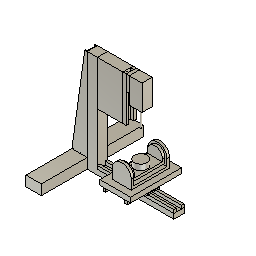
5 Axis CNC Linkage Ideation 3 (Autodesk Fusion 360 design; units mm, degrees)
Autodesk Fusion 360 part; units mm, degrees
sketch "Sketch1" plane through (0, 0, 0) normal (0, 1, 0) x (1, 0, 0)
  line L0 (400, -400) -> (-400, -400)
  line L1 (-400, -400) -> (-400, 400)
  line L2 (-400, 400) -> (400, 400)
  line L3 (400, 400) -> (400, -400)
  line L4 (400, -400) -> (-400, 400) construction
  line L5 (-400, -400) -> (400, 400) construction
  line L6 (-400, -400) -> (-200, -400)
  line L7 (-200, -400) -> (-200, 400)
  line L8 (-200, 400) -> (-400, 400)
  line L9 (-400, 400) -> (-400, -400)
  line L10 (-200, -400) -> (400, -400)
  line L11 (100, -400) -> (100, -50)
  line L12 (100, -50) -> (-200, -50)
  line L13 (200, -400) -> (0, -400)
  line L14 (0, -400) -> (0, -50)
  line L15 (0, -50) -> (200, -50)
  line L16 (200, -50) -> (200, -400)
  line L17 (200, -400) -> (0, -50) construction
  line L18 (0, -400) -> (200, -50) construction
  line L19 (400, 400) -> (-200, 400)
  line L20 (-200, 400) -> (-200, 360)
  line L21 (-200, 360) -> (400, 360)
  line L22 (400, 360) -> (400, 400)
  line L23 (-200, 360) -> (400, 360)
  line L24 (400, 360) -> (400, 335)
  line L25 (400, 335) -> (-200, 335)
  line L26 (-200, 335) -> (-200, 360)
  line L27 (400, 335) -> (-200, 335)
  line L28 (-200, 335) -> (-200, 325)
  line L29 (-200, 325) -> (400, 325)
  line L30 (400, 325) -> (400, 335)
  line L31 (-200, 325) -> (400, 325)
  line L32 (400, 325) -> (400, 300)
  line L33 (400, 300) -> (-200, 300)
  line L34 (-200, 300) -> (-200, 325)
  line L35 (150, -200) -> (50, -200)
  line L36 (50, -200) -> (50, -400)
  line L37 (50, -400) -> (150, -400)
  line L38 (150, -400) -> (150, -200)
  line L39 (150, -200) -> (50, -400) construction
  line L40 (50, -200) -> (150, -400) construction
  line L41 (105, -200) -> (95, -200)
  line L42 (95, -200) -> (95, -50)
  line L43 (95, -50) -> (105, -50)
  line L44 (105, -50) -> (105, -200)
  line L45 (105, -200) -> (95, -50) construction
  line L46 (95, -200) -> (105, -50) construction
  line L47 (175, 260) -> (25, 260)
  line L48 (25, 260) -> (25, 110)
  line L49 (25, 110) -> (175, 110)
  line L50 (175, 110) -> (175, 260)
  line L51 (175, 260) -> (25, 110) construction
  line L52 (25, 260) -> (175, 110) construction
  line L53 (-200, -400) -> (-280, -400)
  line L54 (-280, -400) -> (-280, 400)
  line L55 (-280, 400) -> (-200, 400)
  line L56 (-200, 400) -> (-200, -400)
  line L57 (220, 260) -> (-20, 260)
  line L58 (-20, 260) -> (-20, 300)
  line L59 (-20, 300) -> (220, 300)
  line L60 (220, 300) -> (220, 260)
  line L61 (220, 260) -> (-20, 300) construction
  line L62 (-20, 260) -> (220, 300) construction
  line L63 (25, 300) -> (5, 300)
  line L64 (5, 300) -> (5, 325)
  line L65 (5, 325) -> (25, 325)
  line L66 (25, 325) -> (25, 300)
  line L67 (25, 300) -> (5, 325) construction
  line L68 (5, 300) -> (25, 325) construction
  line L69 (195, 300) -> (175, 300)
  line L70 (175, 300) -> (175, 325)
  line L71 (175, 325) -> (195, 325)
  line L72 (195, 325) -> (195, 300)
  line L73 (195, 300) -> (175, 325) construction
  line L74 (175, 300) -> (195, 325) construction
  line L75 (25, 300) -> (175, 300)
  line L76 (200, 325) -> (0, 325)
  line L77 (0, 325) -> (0, 335)
  line L78 (0, 335) -> (200, 335)
  line L79 (200, 335) -> (200, 325)
  line L80 (200, 325) -> (0, 335) construction
  line L81 (0, 325) -> (200, 335) construction
  line L82 (0, -400) -> (25, -400)
  line L83 (25, -400) -> (25, -50)
  line L84 (25, -50) -> (0, -50)
  line L85 (0, -50) -> (0, -400)
  line L86 (50, -200) -> (25, -200)
  line L87 (25, -200) -> (25, -400)
  line L88 (25, -400) -> (50, -400)
  line L89 (50, -400) -> (50, -200)
  line L90 (25, -400) -> (50, -400)
  line L91 (50, -400) -> (50, -280)
  line L92 (50, -280) -> (25, -280)
  line L93 (25, -280) -> (25, -400)
  line L94 (-280, 400) -> (-400, 400)
  line L95 (-400, 400) -> (-400, 320)
  line L96 (-400, 320) -> (-280, 320)
  line L97 (-280, 320) -> (-280, 400)
  line L98 (25, 260) -> (175, 260)
  line L99 (175, 260) -> (175, 160)
  line L100 (175, 160) -> (25, 160)
  line L101 (25, 160) -> (25, 260)
  point P0 (100, -225)
  point P1 (100, -300)
  point P2 (100, -125)
  point P3 (100, 185)
  point P4 (100, 280)
  point P5 (15, 312.5)
  point P6 (185, 312.5)
  point P7 (100, 330)
  dimension "d1" = 800
  dimension "d2" = 800
  dimension "d3" = 200
  dimension "d4" = 350
  dimension "d5" = 200
  dimension "d6" = 40
  dimension "d7" = 25
  dimension "d8" = 10
  dimension "d9" = 25
  dimension "d10" = 100
  dimension "d11" = 200
  dimension "d12" = 10
  dimension "d13" = 150
  dimension "d14" = 150
  dimension "d15" = 80
  dimension "d21" = 240
  dimension "d22" = 40
  dimension "d27" = 20
  dimension "d28" = 20
  dimension "d29" = 150
  dimension "d30" = 200
  dimension "d41" = 25
  dimension "d46" = 120
  dimension "d55" = 80
  dimension "d73" = 100
  constraint horizontal L0
  constraint perpendicular L0 L1
  constraint parallel L0 L2
  constraint parallel L1 L3
  constraint coincident L4 origin
  constraint coincident L5 origin
  constraint horizontal L6
  constraint vertical L7
  constraint horizontal L8
  constraint vertical L9
  constraint coincident L2 L7.end
  constraint midpoint L10 L11.start
  constraint perpendicular L0 L11
  constraint coincident L7 L12.end
  constraint horizontal L13
  constraint perpendicular L13 L14
  constraint parallel L13 L15
  constraint parallel L14 L16
  constraint coincident L17 P0
  constraint coincident L18 P0
  constraint coincident L10 L13.start
  constraint midpoint L11 P0
  constraint horizontal L19
  constraint vertical L20
  constraint horizontal L21
  constraint vertical L22
  constraint coincident L7 L20.end
  constraint horizontal L23
  constraint vertical L24
  constraint horizontal L25
  constraint vertical L26
  constraint coincident L3 L24.end
  constraint horizontal L27
  constraint vertical L28
  constraint horizontal L29
  constraint vertical L30
  constraint coincident L7 L28.end
  constraint horizontal L31
  constraint vertical L32
  constraint horizontal L33
  constraint vertical L34
  constraint coincident L3 L32.end
  constraint horizontal L35
  constraint perpendicular L35 L36
  constraint parallel L35 L37
  constraint parallel L36 L38
  constraint coincident L39 P1
  constraint coincident L40 P1
  constraint coincident L11 P1
  constraint collinear L0 L37
  constraint horizontal L41
  constraint perpendicular L41 L42
  constraint parallel L41 L43
  constraint parallel L42 L44
  constraint coincident L45 P2
  constraint coincident L46 P2
  constraint coincident L11 P2
  constraint collinear L35 L41
  constraint collinear L15 L43
  constraint horizontal L47
  constraint perpendicular L47 L48
  constraint parallel L47 L49
  constraint parallel L48 L50
  constraint coincident L51 P3
  constraint coincident L52 P3
  constraint horizontal L53
  constraint vertical L54
  constraint horizontal L55
  constraint vertical L56
  constraint collinear L12 L15
  constraint collinear L8 L55
  constraint horizontal L57
  constraint perpendicular L57 L58
  constraint parallel L57 L59
  constraint parallel L58 L60
  constraint coincident L61 P4
  constraint coincident L62 P4
  constraint midpoint L33 L59
  constraint midpoint L47 L57
  constraint horizontal L63
  constraint perpendicular L63 L64
  constraint parallel L63 L65
  constraint parallel L64 L66
  constraint coincident L67 P5
  constraint coincident L68 P5
  constraint collinear L59 L63
  constraint collinear L31 L65
  constraint horizontal L69
  constraint perpendicular L69 L70
  constraint parallel L69 L71
  constraint parallel L70 L72
  constraint coincident L73 P6
  constraint coincident L74 P6
  constraint collinear L29 L71
  constraint collinear L33 L69
  constraint perpendicular L70 L75
  constraint midpoint L33 L75
  constraint horizontal L76
  constraint perpendicular L76 L77
  constraint parallel L76 L78
  constraint parallel L77 L79
  constraint coincident L80 P7
  constraint coincident L81 P7
  constraint midpoint L27 L78
  constraint collinear L31 L76
  constraint horizontal L82
  constraint vertical L83
  constraint horizontal L84
  constraint vertical L85
  constraint coincident L15 L83.end
  constraint horizontal L86
  constraint vertical L87
  constraint horizontal L88
  constraint vertical L89
  constraint horizontal L90
  constraint vertical L91
  constraint horizontal L92
  constraint vertical L93
  constraint coincident L36 L91.end
  constraint horizontal L94
  constraint vertical L95
  constraint horizontal L96
  constraint vertical L97
  constraint coincident L9 L95.end
  constraint horizontal L98
  constraint vertical L99
  constraint horizontal L100
  constraint vertical L101
  constraint coincident L50 L99.end
  measures "d1" distance of L1.end L2.end
  measures "d2" distance of L0.end L1.end
  measures "d3" distance of L0.end L6.end
  measures "d4" distance of L11.start L11.end
  measures "d5" distance of L14.end L15.end
  measures "d6" distance of L2.end L21.end
  measures "d7" distance of L20.end L25.end
  measures "d8" distance of L24.end L29.end
  measures "d9" distance of L28.end L33.end
  measures "d10" distance of L36.end L37.end
  measures "d11" distance of L35.end L36.end
  measures "d12" distance of L42.end L43.end
  measures "d13" distance of L48.end L49.end
  measures "d14" distance of L47.end L48.end
  measures "d15" distance of L6.end L53.end
  measures "d21" distance of L58.end L59.end
  measures "d22" distance of L57.start L59.end
  measures "d27" distance of L64.end L65.end
  measures "d28" distance of L70 L72
  measures "d29" distance of L63.start L69.end
  measures "d30" distance of L77.end L78.end
  measures "d41" distance of L13.end L82.end
  measures "d46" distance of L82.end L92.end
  measures "d55" distance of L54.end L96.end
  measures "d73" distance of L47.end L100.end
extrude "Extrude1" add sketch "Sketch1" along normal mid plane 80 contours L2 L3 L7 L19 L20 L21 L22 L23 L56 | L0 L2 L6 L7 L8 L20 L26 L28 L34 L53 L54 L55 L56 L97 makes body 1
extrude "Extrude2" add sketch "Sketch1" along normal mid plane 80 separate body contours L3 L7 L21 L23 L24 L25 L26 L27 L56 L78 makes body 2
extrude "Extrude3" cut sketch "Sketch1" along normal mid plane 40 contours L3 L7 L21 L23 L24 L25 L26 L27 L56 L78 bodies 2 makes body 3 at (0, 20, -351.6667)
extrude "Extrude4" add sketch "Sketch1" along normal mid plane 100 separate body contours L25 L27 L29 L31 L65 L71 L76 L77 L78 L79 makes body 4
extrude "Extrude5" add sketch "Sketch1" along normal mid plane 400 separate body contours L29 L31 L33 L59 L69 L70 L71 L72 L76 | L29 L31 L33 L59 L63 L64 L65 L66 L76 makes body 5 at (25, 66.6667, -316.6667) makes body 6 at (195, 66.6667, -308.3333)
extrude "Extrude6" add sketch "Sketch1" along normal mid plane 400 separate body contours L33 L47 L57 L58 L59 L60 L63 L69 L75 L98 makes body 7
extrude "Extrude7" add sketch "Sketch1" along normal mid plane 300 separate body contours L47 L48 L50 L57 L98 L99 L100 L101 | L48 L49 L50 L100 makes body 8
extrude "Extrude8" add sketch "Sketch1" along normal mid plane 80 separate body contours L0 L7 L10 L12 L14 L56 L85 makes body 9
extrude "Extrude9" add sketch "Sketch1" along normal mid plane 80 separate body contours L0 L10 L12 L13 L14 L15 L82 L83 L84 L85 L87 L93 makes body 10
extrude "Extrude10" cut sketch "Sketch1" along normal mid plane 40 contours L0 L10 L12 L13 L14 L15 L82 L83 L84 L85 L87 L93 bodies 10 makes body 11 at (16.6667, -40, 166.6667)
extrude "Extrude11" add sketch "Sketch1" along normal mid plane 80 separate body contours L0 L10 L13 L36 L83 L87 L88 L89 L90 L91 L92 L93 makes body 12
extrude "Extrude12" add sketch "Sketch1" along normal mid plane 80 separate body contours L0 L10 L11 L13 L35 L37 L38 L41 | L0 L10 L11 L13 L35 L36 L37 L41 L89 L91 makes body 13
extrude "Extrude13" add sketch "Sketch1" along normal mid plane 10 contours L11 L15 L35 L41 L43 L44 | L11 L12 L15 L35 L41 L42 L43 bodies 13
fillet "Fillet1" radius 5 4 edges at (105, -5, 125) (95, 5, 125) (105, 5, 125) (95, -5, 125) on bodies 13
extrude "Extrude14" add sketch "Sketch1" along normal mid plane 800 separate body contours L1 L2 L8 L9 L54 L94 L95 L96 L97 makes body 14
extrude "Extrude15" add sketch "Sketch1" along normal mid plane 80 separate body contours L0 L1 L6 L9 L54 L96 makes body 15
shell "Shell1" thickness 5 removed faces 2 at (-400, -13.3333, 160) at (-360, 13.3333, 400) on bodies 15
draft "Draft1" angle 8 neutral plane through (-400, 0, -320) pull (0, 0, 1) 1 faces at (-400, 38.3333, -78.3333) on bodies 15
shell "Shell2" thickness 20 removed faces 3 at (25, 50, -160) at (75, -50, -110) at (175, -50, -160) on bodies 8
extrude "Extrude16" add sketch "Sketch1" along normal mid plane 260 separate body contours L47 L48 L50 L57 L98 L99 L100 L101 | L48 L49 L50 L100 makes body 16
combine "Combine1" operation cut target body 16 tool bodies 8 keep tools
fillet "Fillet2" radius 75 4 edges at (175, -140, -110) (175, 140, -110) (25, 140, -110) (25, -140, -110) on bodies 8
move_face "OffsetFaces1" offset -15 4 faces at (125, -43.3333, -240) (175, 43.3333, -153.3333) (75, -43.3333, -110) (25, 43.3333, -196.6667) on bodies 16
shell "Shell4" thickness 20 removed faces 3 at (40, -43.3333, -191.6667) at (120, 43.3333, -125) at (160, -43.3333, -158.3333) on bodies 16
fillet "Fillet3" radius 60 4 edges at (40, 120, -125) (160, 120, -125) (40, -120, -125) (160, -120, -125) on bodies 16
extrude "Extrude17" add sketch "Sketch1" along normal mid plane 100 separate body contours L47 L48 L50 L57 L98 L99 L100 L101 makes body 17
move_face "OffsetFaces2" offset -55 1 faces at (75, 16.6667, -260) on bodies 17
move_face "OffsetFaces3" offset -25 2 faces at (175, 16.6667, -175) (25, 16.6667, -190) on bodies 17
fillet "Fillet4" radius 50 4 edges at (50, 50, -182.5) (150, 50, -182.5) (150, -50, -182.5) (50, -50, -182.5) on bodies 17
